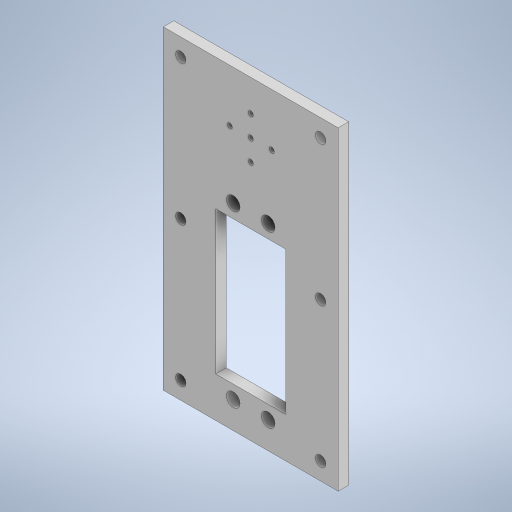
# Autodesk Inventor part: practice_parts01
Saved by Autodesk Inventor 2024.3 (Build 283343000, 343)
## iProperties
Created: 2024-10-22
Part Number: practice_parts01
Material: 一般
Document SubType Name: Modeling
Designer: 佐藤智貴
Density: 1 g/cm^3
Appearance: 既定
Author: 佐藤智貴
Autodesk Inventor part; units mm, degrees
ref_plane "YZ Plane" through (0, 0, 0) normal (1, 0, 0) x (0, 1, 0)
ref_plane "XZ Plane" through (0, 0, 0) normal (0, 1, 0) x (-1, 0, 0)
ref_plane "XY Plane" through (0, 0, 0) normal (0, 0, 1) x (1, 0, 0)
sketch "スケッチ6" plane through (0, 0, 0) normal (0, 0, 1) x (1, 0, 0)
  line L0 (30, 10) -> (30, 100)
  line L1 (30, 100) -> (0, 100)
  line L2 (0, 100) -> (0, 0)
  line L3 (0, 100) -> (-10, 100)
  line L4 (-10, 100) -> (-10, 90)
  line L5 (-10, 90) -> (0, 90)
  line L6 (0, 90) -> (0, 100)
  line L7 (30, 100) -> (40, 100)
  line L8 (40, 100) -> (40, 90)
  line L9 (40, 90) -> (30, 90)
  line L10 (30, 90) -> (30, 100)
  line L11 (0, 50) -> (-10, 50)
  line L12 (-10, 50) -> (-10, 60)
  line L13 (-10, 60) -> (0, 60)
  line L14 (0, 60) -> (0, 50)
  line L15 (30, 50) -> (40, 50)
  line L16 (40, 50) -> (40, 60)
  line L17 (40, 60) -> (30, 60)
  line L18 (30, 60) -> (30, 50)
  line L19 (0, 20) -> (-10, 20)
  line L20 (-10, 20) -> (-10, 10)
  line L21 (-10, 10) -> (0, 10)
  line L22 (0, 10) -> (0, 20)
  line L23 (30, 20) -> (40, 20)
  line L24 (40, 20) -> (40, 10)
  line L25 (40, 10) -> (30, 10)
  line L26 (30, 10) -> (30, 20)
  line L27 (0, 100) -> (30, 100)
  line L28 (30, 100) -> (30, 10)
  line L29 (30, 10) -> (0, 10)
  line L30 (0, 10) -> (0, 100)
  line L31 (-10, 100) -> (40, 100)
  line L32 (40, 100) -> (40, 10)
  line L33 (40, 10) -> (-10, 10)
  line L34 (-10, 10) -> (-10, 100)
  point P0 (0, 90)
  point P1 (30, 55)
  point P2 (0, 10)
  point P3 (0, 10)
  point P4 (0, 60)
  dimension "d73" = 30
  dimension "d117" = 10
  dimension "d118" = 10
  dimension "d119" = 10
  dimension "d120" = 10
  dimension "d141" = 10
  dimension "d142" = 0
  dimension "d143" = 30
  dimension "d144" = 10
  dimension "d145" = 10
  dimension "d146" = 10
  dimension "d147" = 10
  dimension "d149" = 30
  dimension "d167" = 90
  constraints: 70 end point, 17 parallel, 8 horizontal, 8 perpendicular, 6 point on line, 1 midpoint
  measures "d73" distance of L0.end L1.end
  measures "d117" distance of L3.end L4.end
  measures "d118" distance of L4.end L5.end
  measures "d119" distance of L7.end L8.end
  measures "d120" distance of L8.end L9.end
  measures "d141" distance of L15.end L17.start
  measures "d142" distance from line of L0 point (30, 55)
  measures "d143" distance between parallel lines of L9 L17
  measures "d144" distance between parallel lines of L0 L16
  measures "d145" distance between parallel lines of L2 L12
  measures "d146" distance of L19.start L19.end
  measures "d147" distance between parallel lines of L19 L21
  measures "d149" distance between parallel lines of L15 L23
  measures "d167" distance between parallel lines of L29 L1
extrude "押し出し5" add sketch "スケッチ6" along normal blind 3
sketch "スケッチ7" plane through (0, 0, 3) normal (0, 0, 1) x (1, 0, 0)
  line L0 (30, 90) -> (30, 90) projected
  circle A0 centre (15, 85) radius 6
  line L1 (15, 85) -> (15, 104.27)
  line L2 (40, 100) -> (-10, 100) projected
  point P0 (0, 0)
  point P1 (30, 0)
  point P2 (15, 91)
  point P3 (9, 85)
  point P4 (15, 79)
  point P5 (21, 85)
  point P6 (30, 10)
  point P7 (15, 100)
  dimension "d79" = 12
  dimension "d82" = 360
  dimension "d156" = 0
  constraints: 2 end point, 1 coincident, 1 midpoint, 1 point on line, 1 vertical, 1 vertical alignment, 8 other
  measures "d156" distance from line of point (15, 100) L1
hole "穴2" at (15, 85, 3) at (15, 91, 3) at (9, 85, 3) at (15, 79, 3) at (21, 85, 3) direction (0, 0, -1) diameter 1.5 end through all
sketch "スケッチ8" plane through (0, 0, 3) normal (0, 0, 1) x (1, 0, 0)
  line L0 (5, 69) -> (25, 69)
  line L1 (25, 69) -> (25, 15)
  line L2 (25, 15) -> (5, 15)
  line L3 (5, 15) -> (5, 69)
  line L4 (5, 62.45) -> (25, 62.45)
  line L5 (25, 62.45) -> (25, 21.55)
  line L6 (25, 21.55) -> (5, 21.55)
  line L7 (5, 21.55) -> (5, 62.45)
  circle A0 centre (10, 66.3) radius 1.95
  circle A1 centre (20, 66.3) radius 1.95
  circle A2 centre (10, 17.7) radius 1.95
  circle A3 centre (20, 17.7) radius 1.95
  line L8 (-10, 10) -> (40, 10) projected
  line L9 (-10, 100) -> (-10, 10) projected
  point P0 (0, 100)
  point P1 (15, 21.55)
  point P2 (25, 62.45)
  dimension "d91" = 20
  dimension "d93" = 54
  dimension "d96" = 10
  dimension "d98" = 48.6
  dimension "d99" = 2.7
  dimension "d100" = 5
  dimension "d101" = 40.9
  dimension "d102" = 6.55
  dimension "d105" = 3.9
  dimension "d106" = 3.9
  dimension "d107" = 3.9
  dimension "d151" = 3.9
  dimension "d152" = 10
  dimension "d153" = 5
  dimension "d154" = 2.7
  dimension "d168" = 5
  dimension "d169" = 15
  constraints: 16 end point, 4 centre point, 4 parallel, 3 coincident, 2 horizontal, 2 perpendicular, 2 point on line, 1 midpoint
  measures "d91" distance between parallel lines of L1 L3
  measures "d93" distance between parallel lines of L2 L0
  measures "d96" distance of point (20, 66.3) point (10, 66.3)
  measures "d98" distance of point (10, 66.3) point (10, 17.7)
  measures "d99" distance from line of L0 point (20, 66.3)
  measures "d100" distance from line of L1 point (20, 66.3)
  measures "d101" distance from line of point (15, 21.55) L4
  measures "d102" distance between parallel lines of L0 L4
  measures "d105" diameter of A0
  measures "d106" diameter of A1
  measures "d107" diameter of A2
  measures "d151" diameter of A3
  measures "d152" distance of A2.centre A3.centre
  measures "d153" distance from line of L1 A3.centre
  measures "d154" distance from line of L2 A3.centre
  measures "d168" distance between parallel lines of L8 L2
  measures "d169" distance between parallel lines of L9 L7
extrude "押し出し6" cut sketch "スケッチ8" against normal blind 3 contours L4 L1 L6 L3 | A0 | A1 | A2 | A3
sketch "スケッチ9" plane through (0, 0, 3) normal (0, 0, 1) x (1, 0, 0)
  line L0 (-10, 100) -> (-10, 10) projected
  line L1 (40, 90) -> (40, 100) projected
  line L2 (40, 100) -> (-10, 100) projected
  line L3 (0, 60) -> (-10, 60) projected
  line L4 (40, 60) -> (30, 60) projected
  line L5 (40, 50) -> (40, 60) projected
  line L6 (-10, 60) -> (-10, 50) projected
  line L7 (-10, 20) -> (-10, 10) projected
  line L8 (0, 20) -> (-10, 20) projected
  line L9 (40, 20) -> (30, 20) projected
  line L10 (40, 10) -> (40, 20) projected
  point P0 (-5, 95)
  point P1 (35, 95)
  point P2 (-10, 90)
  point P3 (40, 95)
  point P4 (-5, 55)
  point P5 (35, 55)
  point P6 (35, 15)
  point P7 (-5, 15)
  dimension "d126" = 5
  dimension "d127" = 5
  dimension "d157" = 5
  dimension "d158" = 5
  dimension "d159" = 5
  dimension "d160" = 5
  dimension "d161" = 5
  dimension "d162" = 5
  dimension "d163" = 5
  dimension "d164" = 5
  dimension "d165" = 5
  dimension "d166" = 5
  constraints: 1 midpoint
  measures "d126" distance from line of L0 point (-5, 95)
  measures "d127" distance of point (40, 95) point (35, 95)
  measures "d157" distance from line of L2 point (-5, 95)
  measures "d158" distance from line of L2 point (35, 95)
  measures "d159" distance from line of L3 point (-5, 55)
  measures "d160" distance from line of L4 point (35, 55)
  measures "d161" distance from line of L5 point (35, 55)
  measures "d162" distance from line of L6 point (-5, 55)
  measures "d163" distance from line of L7 point (-5, 15)
  measures "d164" distance from line of L8 point (-5, 15)
  measures "d165" distance from line of L9 point (35, 15)
  measures "d166" distance from line of L10 point (35, 15)
hole "穴3" at (-5, 95, 3) at (35, 95, 3) at (-5, 55, 3) at (35, 55, 3) at (35, 15, 3) at (-5, 15, 3) direction (0, 0, -1) diameter 3 end through all
equation "\"d120\" = d119"
equation "\"d141\" = d120"
equation "\"d144\" = d120"
equation "\"d145\" = d144"
equation "\"d147\" = d141"
equation "\"d149\" = d143"
equation "\"d98\" = d95"
equation "\"d151\" = d107"
equation "\"d127\" = d126"
equation "\"d159\" = d157"
equation "\"d160\" = d159"
equation "\"d164\" = d163"
equation "\"d165\" = d164"
equation "\"d95\" = 48.6"
